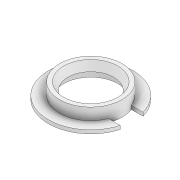
# Autodesk Inventor part: Sujección_piezas_sonar
Saved by Autodesk Inventor 2022.3 (Build 263350000, 350)
## iProperties
Created: 2023-07-18
Part Number: Sujección_piezas_sonar
Material: Genérico
Document SubType Name: Modeling
Designer: Usuario
Density: 1 g/cm^3
Appearance: Valor por defecto
Author: Usuario
Autodesk Inventor part; units mm, degrees
ref_plane "YZ Plane" through (0, 0, 0) normal (1, 0, 0) x (0, 1, 0)
ref_plane "XZ Plane" through (0, 0, 0) normal (0, 1, 0) x (-1, 0, 0)
ref_plane "XY Plane" through (0, 0, 0) normal (0, 0, 1) x (1, 0, 0)
sketch "Boceto1" plane through (0, 0, 0) normal (0, 1, 0) x (-1, 0, 0)
  circle A0 centre (0, 0) radius 18
  circle A1 centre (0, 0) radius 9.75
  dimension "d0" = 36
  dimension "d1" = 19.5
  constraints: 2 centre point, 2 coincident
  measures "d0" diameter of A0
  measures "d1" diameter of A1
extrude "Extrusión1" add sketch "Boceto1" along normal blind 1.5
sketch "Boceto2" plane through (0, 1.5, 0) normal (0, 1, 0) x (1, 0, 0)
  circle A0 centre (0, 0) radius 9.75
  circle A1 centre (0, 0) radius 13.25
  dimension "d4" = 26.5
  constraints: 2 centre point, 2 coincident
  measures "d4" diameter of A1
extrude "Extrusión2" add sketch "Boceto2" along normal blind 5
sketch "Boceto3" plane through (0, 1.5, 0) normal (0, 1, 0) x (1, 0, 0)
  circle A0 centre (0, 0) radius 18 projected
  line L0 (18, 0) -> (18, -4.85)
  line L1 (18, -4.85) -> (12.3305, -4.85)
  circle A1 centre (0, 0) radius 13.25 projected
  line L2 (18, 0) -> (18, 4.85)
  line L3 (18, 4.85) -> (12.3305, 4.85)
  point P0 (17.3343, 4.85)
  point P1 (17.3343, -4.85)
  dimension "d7" = 4.85
  dimension "d8" = 4.85
  constraints: 8 end point, 3 perpendicular, 3 vertical, 2 point on circle, 2 other
  measures "d7" distance of L0.start L0.end
  measures "d8" distance of L0.start L2.end
extrude "Extrusión3" cut sketch "Boceto3" against normal through all contours A0 L1 A1 L3 picked at (14.5628, -2.7275)
sketch "Boceto4" plane through (0, 0, 0) normal (0, 0, 1) x (1, 0, 0)
  line L0 (9.75, 6.5) -> (9.75, 0) projected
  line L1 (13.25, 0) -> (13.25, 6.5) projected
  line L2 (13.25, 6.5) -> (9.75, 6.5)
  line L3 (11.5, 6.5) -> (9.75, 3.25)
  line L4 (9.75, 3.25) -> (11.5, 0)
  line L5 (17.3343, 0) -> (-18, 0) projected
  line L6 (11.5, 0) -> (13.25, 0)
  line L7 (11.5, 0) -> (9.75, 0)
  line L8 (9.75, 0) -> (9.75, 6.5)
  line L9 (9.75, 6.5) -> (11.5, 6.5)
  line L10 (13.25, 6.5) -> (-13.25, 6.5) projected
  point P0 (0, 0)
  constraints: 14 end point, 3 perpendicular, 2 midpoint, 1 collinear, 1 parallel, 1 point on line
sketch3d "Boceto 3D1"
  arc A0 (9.75, 6.5, 0) -> (0, 6.5, 9.75) centre (0, 6.5, 0) ccw
  arc A1 (0, 6.5, 9.75) -> (-9.75, 6.5, 0) centre (0, 6.5, 0) ccw
  arc A2 (-9.75, 6.5, 0) -> (0, 6.5, -9.75) centre (0, 6.5, 0) ccw
  arc A3 (0, 6.5, -9.75) -> (9.75, 6.5, 0) centre (0, 6.5, 0) ccw
sweep "Barrido1" cut profiles "Boceto4" path "Boceto 3D1" contours L2 L3 L0 | L4 L5 L0
